Autodesk Fusion 360 part; units mm, degrees
note: some values were not read from the file. Chosen so that the rebuilt part matches the saved one: which bodies a step acts on; which face or edge a step refers to.
(part 2 of 2)
equation "d220 = frame_profile"
equation "d232 = hole"
equation "d244 = hole"
equation "d249 = hole"
equation "d252 = frame_profile"
equation "d256 = hole"
equation "d283 = hole"
named bodies: "profile", "profile (12)", "profile (14)", "profile (4)", "profile (1)", "profile (2)", "profile (9)", "profile (10)", "profile (15)", "profile (13)", "profile (3)", "profile (16)", "profile (5)", "profile (6)", "profile (8)", "profile (7)", "profile (11)", "profile (17)", "profile (18)", "profile (9) (1)", "profile (9) (2)"
